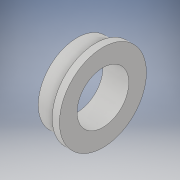
# Autodesk Inventor part: ActoBotics Bearing .375
Saved by Autodesk Inventor 2017 (Build 210142000, 142)
## iProperties
Created: 2017-08-25
Part Number: ActoBotics Bearing .375
Material: Generic
Document SubType Name: Modeling
Designer: Austin M.
Density: 1 g/cm^3
Appearance: Default
Author: Austin M.
Autodesk Inventor part; units mm, degrees
ref_plane "YZ Plane" through (0, 0, 0) normal (1, 0, 0) x (0, 1, 0)
ref_plane "XZ Plane" through (0, 0, 0) normal (0, 1, 0) x (-1, 0, 0)
ref_plane "XY Plane" through (0, 0, 0) normal (0, 0, 1) x (1, 0, 0)
sketch "Sketch1" plane through (0, 0, 0) normal (0, 0, 1) x (1, 0, 0)
  line L0 (0, 0) -> (2.4121, 0)
  line L1 (3.175, 3.175) -> (0, 3.175)
  line L2 (0, 3.175) -> (0, 4.7625)
  line L3 (0, 4.7625) -> (2.286, 4.7625)
  line L4 (2.286, 4.7625) -> (2.286, 5.334)
  line L5 (2.286, 5.334) -> (3.175, 5.334)
  line L6 (3.175, 5.334) -> (3.175, 3.175)
  dimension "d0" = 6.35
  dimension "d1" = 9.525
  dimension "d2" = 10.668
  dimension "d3" = 2.286
  dimension "d4" = 0.889
  constraints: 14 end point, 5 perpendicular, 2 horizontal, 1 vertical alignment
  measures "d0" diameter of L1 L0
  measures "d1" diameter of L3 L0
  measures "d2" diameter of L5 L0
  measures "d3" distance of L2.end L3.end
  measures "d4" distance of L4.end L5.end
revolve "Revolution1" add sketch "Sketch1" angle 360 about axis through (0, 0, 0) along (1, 0, 0)
body "Solid1"
